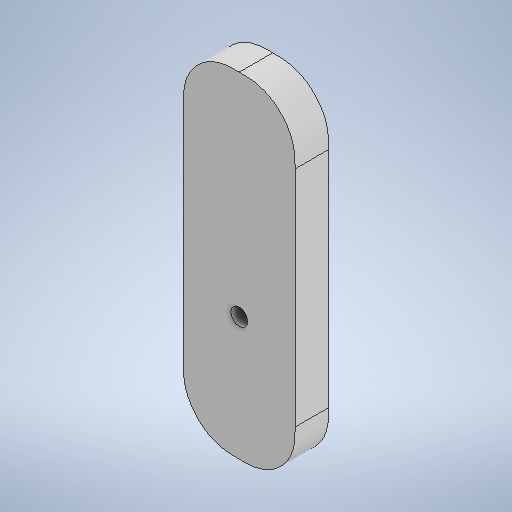
# Autodesk Inventor part: BigServoEjectorArm
Saved by Autodesk Inventor 2025.1 (Build 291241000, 241)
## iProperties
Created: 2025-02-24
Part Number: BigServoEjectorArm
Material: Generic
Document SubType Name: Modeling
Designer: 13156
Density: 1 g/cm^3
Appearance: Default
Author: 13156
Autodesk Inventor part; units mm, degrees
ref_plane "YZ Plane" through (0, 0, 0) normal (1, 0, 0) x (0, 1, 0)
ref_plane "XZ Plane" through (0, 0, 0) normal (0, 1, 0) x (-1, 0, 0)
ref_plane "XY Plane" through (0, 0, 0) normal (0, 0, 1) x (1, 0, 0)
sketch "Sketch1" plane through (0, 0, 0) normal (0, 0, 1) x (1, 0, 0)
  circle A0 centre (-0.0321, 17.0037) radius 0.85
  circle A1 centre (-0.0321, -17.1963) radius 0.85
  line L0 (-0.0321, -0.0963) -> (-0.0321, 17.0037) construction
  line L1 (-0.0321, -17.1963) -> (-0.0321, -0.0963) construction
  circle A2 centre (-0.0321, 17.0037) radius 2.65
  circle A3 centre (-0.0321, -17.1963) radius 2.65
  circle A4 centre (-0.0321, -0.0963) radius 6
  line L2 (-2.6591, -17.5447) -> (-4.4321, -4.1755)
  line L3 (4.3679, -4.1755) -> (2.5949, -17.5447)
  line L4 (-4.4321, 3.9829) -> (-2.6591, 17.3521)
  line L5 (2.5949, 17.3521) -> (4.3679, 3.9829)
  circle A5 centre (-0.0321, -0.0963) radius 1.5
  circle A6 centre (-0.0321, -0.0963) radius 4
  line L6 (9.9679, 37.8037) -> (-10.0321, 37.8037)
  line L7 (-10.0321, 37.8037) -> (-10.0321, -22.1963)
  line L8 (-10.0321, -22.1963) -> (9.9679, -22.1963)
  line L9 (9.9679, -22.1963) -> (9.9679, 37.8037)
  point P0 (0, 0)
  dimension "d0" = 1.7
  dimension "d1" = 1.7
  dimension "d2" = 17.1
  dimension "d3" = 5.3
  dimension "d4" = 5.3
  dimension "d5" = 12
  dimension "d6" = 8.8
  dimension "d7" = 8.8
  dimension "d8" = 3
  dimension "d9" = 8
  dimension "d10" = 5
  dimension "d11" = 60
  dimension "d12" = 20
  constraints: 20 end point, 8 point on circle, 7 centre point, 5 coincident, 4 tangent, 3 equal length, 2 parallel, 1 collinear, 1 horizontal, 1 perpendicular, 1 vertical, 1 other
  measures "d0" diameter of A1
  measures "d1" diameter of A0
  measures "d2" distance of L0.start L0.end
  measures "d3" diameter of A2
  measures "d4" diameter of A3
  measures "d5" diameter of A4
  measures "d6" distance of L5.end L4.start
  measures "d7" distance of L3.start L2.end
  measures "d8" diameter of A5
  measures "d9" diameter of A6
  measures "d10" distance from line of L8 L1.start
  measures "d11" distance between parallel lines of L8 L6
  measures "d12" distance between parallel lines of L7 L9
extrude "Extrusion1" add sketch "Sketch1" along normal blind 6 contours A0 | A1 | A2 | A2 L5 A4 L4 | A4 | A4 L3 A3 L2 | A3 | A5 | A6 | L9 L8 L7 L6
extrude "Extrusion2" cut sketch "Sketch1" along normal blind 2.5 contours A0 | A1 | A2 | A2 L5 A4 L4 | A4 | A4 L3 A3 L2 | A3 | A5 | A6
extrude "Extrusion3" cut sketch "Sketch1" along normal blind 6 contours A5
fillet "Fillet1" radius 10 4 edges at (9.9679, 37.8037, 3) (-10.0321, 37.8037, 3) (9.9679, -22.1963, 3) (-10.0321, -22.1963, 3) curvature continuous yes
equation "\"d4\" = d3"
equation "\"d7\" = d6"
body "Solid1"
